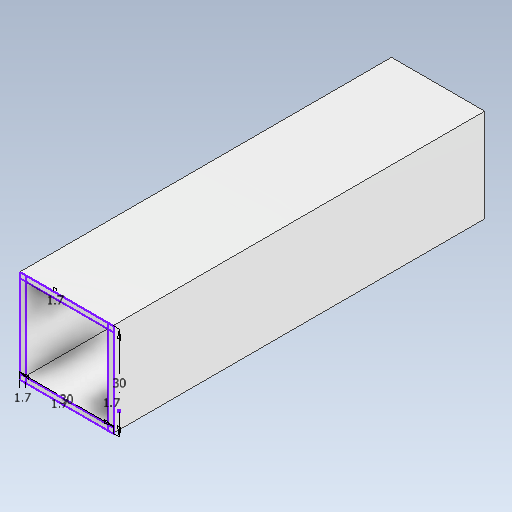
# Autodesk Inventor part: Cablecanal Ranurado 30x30 L=115  mm
Saved by Autodesk Inventor 2020 (Build 240168000, 168)
## iProperties
Created: 2020-09-30
Part Number: Cablecanal Ranurado 30x30 L=115  mm
Material: PVC-Piping
Document SubType Name: Modeling
Designer: Hernan
Density: 1.4 g/cm^3
Appearance: Smooth - White
Author: Hernan
Autodesk Inventor part; units mm, degrees
ref_plane "YZ Plane" through (0, 0, 0) normal (1, 0, 0) x (0, 1, 0)
ref_plane "XZ Plane" through (0, 0, 0) normal (0, 1, 0) x (-1, 0, 0)
ref_plane "XY Plane" through (0, 0, 0) normal (0, 0, 1) x (1, 0, 0)
sketch "Sketch1" plane through (0, 0, 0) normal (0, 0, 1) x (1, 0, 0)
  line L0 (-31.9903, -7.2804) -> (-1.9903, -7.2804)
  line L1 (-1.9903, -7.2804) -> (-1.9903, 22.7196)
  line L2 (-1.9903, 22.7196) -> (-31.9903, 22.7196)
  line L3 (-31.9903, -7.2804) -> (-31.9903, 22.7196)
  line L4 (-30.2903, 22.7196) -> (-30.2903, -7.2804)
  line L5 (-31.9903, -5.5804) -> (-1.9903, -5.5804)
  line L6 (-3.6903, 22.7196) -> (-3.6903, -7.2804)
  line L7 (-31.9903, 21.0196) -> (-1.9903, 21.0196)
  point P0 (0, 0)
  point P1 (0, 0)
  point P2 (-3.6903, 21.0196)
  point P3 (-30.2903, 21.0196)
  point P4 (-30.2903, -5.5804)
  point P5 (-3.6903, -5.5804)
  dimension "d0" = 30
  dimension "d1" = 30
  dimension "d2" = 1.7
  dimension "d3" = 1.7
  dimension "d4" = 1.7
  dimension "d5" = 1.7
  constraints: 16 end point, 8 point on line, 3 horizontal, 2 perpendicular, 2 vertical, 1 parallel
  measures "d0" distance of L0.start L0.end
  measures "d1" distance of L0.end L1.end
  measures "d2" distance between parallel lines of L0 L5
  measures "d3" distance between parallel lines of L3 L4
  measures "d4" distance between parallel lines of L1 L6
  measures "d5" distance between parallel lines of L2 L7
extrude "Extrusion1" add sketch "Sketch1" against normal blind 119.543
extrude "Extrusion2" cut sketch "Sketch1" against normal blind 119.543 contours L4 L7 L6 L5
body "Solid1"
